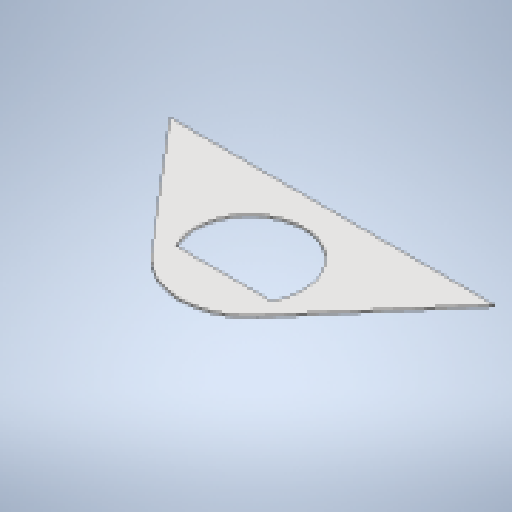
# Autodesk Inventor part: ДМФ 054 фланец лотка v2.0
Saved by Autodesk Inventor 2026.2 (Build 302298000, 298)
## iProperties
Created: 2024-05-14
Part Number: ДМФ 054 фланец лотка v2.0
Material: Generic
Document SubType Name: Sheet Metal
Designer: admin
Density: 1 g/cm^3
Sheet Metal Rule: Default_mm
Appearance: Default
Mass: 10.0564 g
Surface Area: 111.42 cm^2
Volume: 10.0564 cm^3
Flat Pattern Width: 14.75 cm
Flat Pattern Length: 31.5 cm
Flat Pattern Area: 464.625 cm^2
Sheet Metal Width: 147,500 mm
Sheet Metal Length: 315,000 mm
Sheet Metal Area: 46462,500 mm^2
Author: admin
Autodesk Inventor part; units mm, degrees
ref_plane "YZ Plane" through (0, 0, 0) normal (1, 0, 0) x (0, 1, 0)
ref_plane "XZ Plane" through (0, 0, 0) normal (0, 1, 0) x (-1, 0, 0)
ref_plane "XY Plane" through (0, 0, 0) normal (0, 0, 1) x (1, 0, 0)
sketch "Sketch2" plane through (0, 0, 0) normal (0, 0, 1) x (1, 0, 0)
  circle A0 centre (0, 0) radius 67.5
  line L0 (-157.5, 80) -> (-51.2445, -43.9346)
  line L1 (157.5, 80) -> (51.2445, -43.9346)
  line L2 (-157.5, 80) -> (157.5, 80)
  circle A1 centre (0, 0) radius 52.5
  line L3 (46.1655, -25) -> (-46.1655, -25)
  point P0 (0, 80)
  dimension "d11" = 135
  dimension "d12" = 15
  dimension "d13" = 315
  dimension "d14" = 80
  dimension "d15" = 25
  measures "d11" diameter of A0
  measures "d12" radial gap between concentric circles of A0 A1
  measures "d13" distance of L1.start L0.start
  measures "d14" distance from line of point (0, 0) L2
  measures "d15" distance from line of L3 point (0, 0)
extrude "Plate2" add sketch "Sketch2" along normal blind 2 contours A0 | A0 L0 L2 L1 | L3 A1 picked at (-3.1172, -43.6181)
equation "\"d10\" = Thickness"
equation "\"BendRadius\" = Thickness"
equation "\"BendReliefWidth\" = Thickness"
equation "\"BendReliefDepth\" = 0.5 * Thickness"
equation "\"CornerReliefSize\" = 4 * Thickness"
equation "\"MinimumRemnant\" = 2 * Thickness"
equation "\"TransitionRadius\" = BendRadius"
equation "\"JacobiRadiusSize\" = BendRadius"
equation "\"GapSize\" = Thickness"
equation "\"Thickness\" = 2"
body "Solid2"
